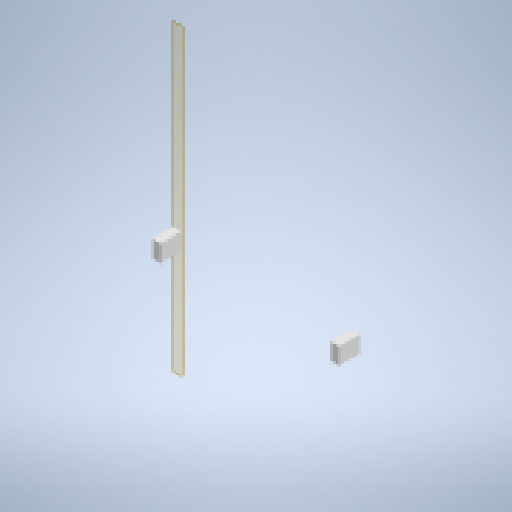
# Autodesk Inventor part: Stand
Saved by Autodesk Inventor 2024 (Build 280153000, 153)
## iProperties
Created: 2024-04-16
Part Number: Stand
Material: Generic
Document SubType Name: Modeling
Designer: teeta
Density: 1 g/cm^3
Appearance: Default
Author: teeta
Autodesk Inventor part; units mm, degrees
ref_plane "YZ Plane" through (0, 0, 0) normal (1, 0, 0) x (0, 1, 0)
ref_plane "XZ Plane" through (0, 0, 0) normal (0, 1, 0) x (-1, 0, 0)
ref_plane "XY Plane" through (0, 0, 0) normal (0, 0, 1) x (1, 0, 0)
ref_plane "Work Plane1" through (-838.1, 1200, 0) normal (0, 0, 1) x (-1, 0, 0)
sketch "Sketch1" plane through (-838.1, 1200, 0) normal (0, 0, 1) x (-1, 0, 0)
  line L0 (0, 792.7005) -> (-38.1, 792.7005)
  line L1 (-38.1, 792.7005) -> (-38.1, 717.8512)
  line L2 (-38.1, 717.8512) -> (0, 717.8512)
  line L3 (0, 717.8512) -> (0, 792.7005)
  line L4 (0, 1219.05) -> (0, -19.05) projected
  line L5 (-38.1, 1180.95) -> (-38.1, 19.05) projected
  line L6 (-838.1, 1219.05) -> (0, 1219.05) construction
  line L7 (-419.05, 1219.05) -> (-419.05, -161.3247) construction
  line L8 (-838.1, 792.7005) -> (-800, 792.7005)
  line L9 (-800, 792.7005) -> (-800, 717.8512)
  line L10 (-800, 717.8512) -> (-838.1, 717.8512)
  line L11 (-838.1, 717.8512) -> (-838.1, 792.7005)
  point P0 (-838.1, 1200)
  constraints: 18 end point, 4 symmetric about line, 2 collinear, 2 parallel, 1 horizontal, 1 midpoint, 1 perpendicular, 1 vertical
extrude "Extrusion1" add sketch "Sketch1" along normal blind 30
sketch "Sketch3" plane through (0, 407.2995, 0) normal (1, 0, 0) x (0, 0, -1)
  line L0 (0, 0) -> (-30, 0) projected
  line L1 (0, 0) -> (-15, 0)
  line L2 (-15, 0) -> (-15, 20.0711)
  arc A0 (-15, 54.7782) -> (-15, 20.0711) centre (-12.4618, 37.4246) ccw
  line L3 (-30, 0) -> (-30, 74.8493) projected
  line L4 (0, 0) -> (0, 74.8493) projected
  line L5 (0, 37.4246) -> (-30, 37.4246) construction
  line L6 (-15, 74.8493) -> (-15, 54.7782)
  line L7 (0, 74.8493) -> (-30, 74.8493) projected
  line L8 (-15, 74.8493) -> (0, 74.8493) construction
  line L9 (0, 74.8493) -> (0, 0) construction
  circle A1 centre (-12.4618, 37.4246) radius 10
  line L10 (-15, 74.8493) -> (0, 74.8493)
  point P0 (0, -407.2995)
  point P1 (-30, 37.4246)
  dimension "d5" = 20
  dimension "d6" = 17.5382
  dimension "d7" = 15
  constraints: 14 end point, 3 midpoint, 2 centre point, 2 perpendicular, 2 point on circle, 1 coincident, 1 collinear, 1 point on line, 1 symmetric about line, 1 tangent, 1 vertical
  measures "d5" diameter of A1
  measures "d6" radius of A0
  measures "d7" distance of L0.start L1.end
extrude "Extrusion3" cut sketch "Sketch3" against normal through all contours L0 L3 A0 L2 | L6 A0 L3 L7 | A1
body "Solid1"
